Autodesk Fusion 360 part; units mm, degrees
note: some values were not read from the file. Set by a fixed rule: which sketch regions a step uses.
(part 2 of 8)
  line L93 (183.7882, -189.4826) -> (184.4852, -189.4634)
  spline S326 degree 3 poles (184.4852, -189.4634) (184.503, -190.2023) (184.6781, -192.2532) (184.527, -192.5784) knots 0 0 0 0 1 1 1 1
  spline S327 degree 3 poles (184.527, -192.5784) (183.4311, -191.7836) (182.2603, -193.7085) (183.3586, -193.8838) knots 0 0 0 0 1 1 1 1
  spline S328 degree 3 poles (183.3586, -193.8838) (183.8477, -193.9337) (184.1665, -193.9552) (184.6949, -194.0483) knots 0 0 0 0 1 1 1 1
  spline S329 degree 2 poles (184.6949, -194.0483) (184.7596, -194.5248) (184.7763, -194.8358) knots 0 0 0 1 1 1
  spline S330 degree 3 poles (184.7763, -194.8358) (183.9042, -195.3624) (183.4164, -195.9409) (183.2408, -196.7861) knots 0 0 0 0 1 1 1 1
  spline S331 degree 3 poles (183.2408, -196.7861) (183.1875, -197.6071) (183.7053, -198.7877) (184.6749, -199.0522) knots 0 0 0 0 1 1 1 1
  line L94 (184.6749, -199.0522) -> (184.423, -200.3759)
  spline S332 degree 3 poles (184.423, -200.3759) (183.7928, -200.5585) (183.5709, -200.5779) (182.9409, -200.6201) knots 0 0 0 0 1 1 1 1
  spline S333 degree 3 poles (182.9409, -200.6201) (182.6208, -200.6492) (182.7483, -200.87) (182.8157, -201.1544) knots 0 0 0 0 1 1 1 1
  spline S334 degree 3 poles (182.8157, -201.1544) (182.9162, -201.4784) (182.7891, -201.5678) (183.1468, -201.7487) knots 0 0 0 0 1 1 1 1
  spline S335 degree 3 poles (183.1468, -201.7487) (183.464, -201.8608) (183.6385, -201.9315) (183.9663, -202.1236) knots 0 0 0 0 1 1 1 1
  spline S336 degree 3 poles (183.9663, -202.1236) (183.9935, -202.4344) (183.976, -202.8518) (184.007, -203.1742) knots 0 0 0 0 1 1 1 1
  spline S337 degree 3 poles (184.007, -203.1742) (184.1755, -203.8454) (184.5886, -204.0182) (185.3208, -203.949) knots 0 0 0 0 1 1 1 1
  spline S338 degree 3 poles (185.3208, -203.949) (186.1138, -203.6409) (186.3928, -203.0862) (186.4441, -202.4283) knots 0 0 0 0 1 1 1 1
  spline S339 degree 2 poles (186.4441, -202.4283) (186.5431, -199.3372) (186.4347, -198.0017) knots 0 0 0 1 1 1
  line L95 (186.4347, -198.0017) -> (185.4047, -196.9892)
  line L96 (185.4047, -196.9892) -> (186.6001, -195.8305)
  spline S340 degree 3 poles (186.6001, -195.8305) (186.3828, -191.254) (186.2731, -187.3174) (185.6278, -182.7417) knots 0 0 0 0 1 1 1 1
  spline S341 degree 3 poles (185.6278, -182.7417) (185.4537, -182.1579) (185.066, -181.8566) (184.4242, -181.7632) knots 0 0 0 0 1 1 1 1
  spline S342 degree 3 poles (160.4078, -156.8007) (157.9023, -157.1956) (155.5538, -158.6101) (153.958, -160.6852) knots 0 0 0 0 1 1 1 1
  spline S343 degree 3 poles (153.958, -160.6852) (152.3623, -162.7604) (151.535, -165.476) (151.686, -168.1431) knots 0 0 0 0 1 1 1 1
  spline S344 degree 3 poles (151.686, -168.1431) (151.829, -170.6692) (152.8449, -173.1304) (154.5006, -174.962) knots 0 0 0 0 1 1 1 1
  spline S345 degree 3 poles (154.5006, -174.962) (156.1564, -176.7936) (158.4388, -177.9812) (160.8245, -178.2524) knots 0 0 0 0 1 1 1 1
  line L97 (160.8245, -178.2524) -> (169.7689, -178.3081)
  spline S346 degree 3 poles (169.7689, -178.3081) (173.9803, -176.478) (178.5319, -175.5232) (183.0868, -175.5142) knots 0 0 0 0 1 1 1 1
  spline S347 degree 3 poles (183.0868, -175.5142) (188.9607, -175.5026) (194.8313, -177.0765) (199.9869, -180.0452) knots 0 0 0 0 1 1 1 1
  line L98 (199.9869, -180.0452) -> (207.8706, -180.5328)
  spline S348 degree 3 poles (207.8706, -180.5328) (210.513, -180.3699) (213.0767, -179.0716) (214.8493, -176.9985) knots 0 0 0 0 1 1 1 1
  spline S349 degree 3 poles (214.8493, -176.9985) (216.622, -174.9255) (217.5826, -172.1023) (217.4642, -169.3136) knots 0 0 0 0 1 1 1 1
  spline S350 degree 3 poles (217.4642, -169.3136) (217.3685, -167.0606) (216.5801, -164.8462) (215.246, -163.0838) knots 0 0 0 0 1 1 1 1
  spline S351 degree 3 poles (215.246, -163.0838) (213.912, -161.3214) (212.0391, -160.02) (209.9773, -159.4225) knots 0 0 0 0 1 1 1 1
  line L99 (209.9773, -159.4225) -> (201.3192, -158.7839)
  spline S352 degree 3 poles (201.3192, -158.7839) (196.2891, -161.1841) (190.713, -162.2999) (185.1988, -162.0098) knots 0 0 0 0 1 1 1 1
  spline S353 degree 3 poles (185.1988, -162.0098) (179.7817, -161.7247) (174.433, -160.084) (169.716, -157.2605) knots 0 0 0 0 1 1 1 1
  line L100 (169.716, -157.2605) -> (160.4078, -156.8007)
  spline S354 degree 3 poles (158.3675, -159.7622) (158.1166, -159.7544) (157.8633, -159.8596) (157.6892, -160.0503) knots 0 0 0 0 1 1 1 1
  spline S355 degree 3 poles (157.6892, -160.0503) (157.5151, -160.241) (157.4245, -160.5147) (157.4538, -160.7776) knots 0 0 0 0 1 1 1 1
  spline S356 degree 3 poles (157.4538, -160.7776) (157.4812, -161.0245) (157.613, -161.2554) (157.804, -161.401) knots 0 0 0 0 1 1 1 1
  spline S357 degree 3 poles (157.804, -161.401) (157.9951, -161.5465) (158.2421, -161.6059) (158.475, -161.5674) knots 0 0 0 0 1 1 1 1
  spline S358 degree 3 poles (158.475, -161.5674) (158.6793, -161.5335) (158.8726, -161.4252) (159.0102, -161.2623) knots 0 0 0 0 1 1 1 1
  spline S359 degree 3 poles (159.0102, -161.2623) (159.1479, -161.0995) (159.2281, -160.8829) (159.2275, -160.6648) knots 0 0 0 0 1 1 1 1
  spline S360 degree 3 poles (159.2275, -160.6648) (159.2267, -160.429) (159.1308, -160.1961) (158.9712, -160.0309) knots 0 0 0 0 1 1 1 1
  spline S361 degree 3 poles (158.9712, -160.0309) (158.8116, -159.8658) (158.5909, -159.7694) (158.3675, -159.7622) knots 0 0 0 0 1 1 1 1
  spline S362 degree 3 poles (157.7617, -173.0749) (157.5108, -173.0671) (157.2574, -173.1722) (157.0833, -173.363) knots 0 0 0 0 1 1 1 1
  spline S363 degree 3 poles (157.0833, -173.363) (156.9092, -173.5536) (156.8187, -173.8274) (156.8479, -174.0903) knots 0 0 0 0 1 1 1 1
  spline S364 degree 3 poles (156.8479, -174.0903) (156.8753, -174.3372) (157.0071, -174.5681) (157.1982, -174.7136) knots 0 0 0 0 1 1 1 1
  spline S365 degree 3 poles (157.1982, -174.7136) (157.3893, -174.8592) (157.6363, -174.9186) (157.8692, -174.88) knots 0 0 0 0 1 1 1 1
  spline S366 degree 3 poles (157.8692, -174.88) (158.0735, -174.8462) (158.2667, -174.7378) (158.4044, -174.575) knots 0 0 0 0 1 1 1 1
  spline S367 degree 3 poles (158.4044, -174.575) (158.542, -174.4121) (158.6223, -174.1956) (158.6216, -173.9774) knots 0 0 0 0 1 1 1 1
  spline S368 degree 3 poles (158.6216, -173.9774) (158.6209, -173.7417) (158.525, -173.5087) (158.3654, -173.3436) knots 0 0 0 0 1 1 1 1
  spline S369 degree 3 poles (158.3654, -173.3436) (158.2058, -173.1785) (157.9851, -173.0821) (157.7617, -173.0749) knots 0 0 0 0 1 1 1 1
  spline S370 degree 3 poles (174.2321, -167.2173) (173.9813, -167.2095) (173.7279, -167.3147) (173.5538, -167.5054) knots 0 0 0 0 1 1 1 1
  spline S371 degree 3 poles (173.5538, -167.5054) (173.3797, -167.6961) (173.2892, -167.9698) (173.3184, -168.2327) knots 0 0 0 0 1 1 1 1
  spline S372 degree 3 poles (173.3184, -168.2327) (173.3458, -168.4796) (173.4776, -168.7105) (173.6687, -168.856) knots 0 0 0 0 1 1 1 1
  spline S373 degree 3 poles (173.6687, -168.856) (173.8597, -169.0016) (174.1068, -169.061) (174.3396, -169.0224) knots 0 0 0 0 1 1 1 1
  spline S374 degree 3 poles (174.3396, -169.0224) (174.544, -168.9886) (174.7372, -168.8802) (174.8749, -168.7174) knots 0 0 0 0 1 1 1 1
  spline S375 degree 3 poles (174.8749, -168.7174) (175.0125, -168.5546) (175.0928, -168.338) (175.0921, -168.1199) knots 0 0 0 0 1 1 1 1
  spline S376 degree 3 poles (175.0921, -168.1199) (175.0913, -167.8841) (174.9955, -167.6511) (174.8359, -167.486) knots 0 0 0 0 1 1 1 1
  spline S377 degree 3 poles (174.8359, -167.486) (174.6763, -167.3209) (174.4556, -167.2245) (174.2321, -167.2173) knots 0 0 0 0 1 1 1 1
  spline S378 degree 3 poles (194.916, -168.2945) (194.6651, -168.2867) (194.4117, -168.3919) (194.2376, -168.5826) knots 0 0 0 0 1 1 1 1
  spline S379 degree 3 poles (194.2376, -168.5826) (194.0636, -168.7733) (193.973, -169.047) (194.0022, -169.3099) knots 0 0 0 0 1 1 1 1
  spline S380 degree 3 poles (194.0022, -169.3099) (194.0297, -169.5568) (194.1615, -169.7877) (194.3525, -169.9333) knots 0 0 0 0 1 1 1 1
  spline S381 degree 3 poles (194.3525, -169.9333) (194.5436, -170.0788) (194.7906, -170.1382) (195.0235, -170.0997) knots 0 0 0 0 1 1 1 1
  spline S382 degree 3 poles (195.0235, -170.0997) (195.2278, -170.0658) (195.4211, -169.9575) (195.5587, -169.7946) knots 0 0 0 0 1 1 1 1
  spline S383 degree 3 poles (195.5587, -169.7946) (195.6964, -169.6318) (195.7766, -169.4153) (195.776, -169.1971) knots 0 0 0 0 1 1 1 1
  spline S384 degree 3 poles (195.776, -169.1971) (195.7752, -168.9613) (195.6793, -168.7284) (195.5197, -168.5632) knots 0 0 0 0 1 1 1 1
  spline S385 degree 3 poles (195.5197, -168.5632) (195.3601, -168.3981) (195.1394, -168.3017) (194.916, -168.2945) knots 0 0 0 0 1 1 1 1
  spline S386 degree 3 poles (211.3226, -162.5043) (211.0718, -162.4965) (210.8184, -162.6017) (210.6443, -162.7924) knots 0 0 0 0 1 1 1 1
  spline S387 degree 3 poles (210.6443, -162.7924) (210.4702, -162.9831) (210.3796, -163.2568) (210.4089, -163.5197) knots 0 0 0 0 1 1 1 1
  spline S388 degree 3 poles (210.4089, -163.5197) (210.4363, -163.7666) (210.5681, -163.9975) (210.7592, -164.143) knots 0 0 0 0 1 1 1 1
  spline S389 degree 3 poles (210.7592, -164.143) (210.9502, -164.2886) (211.1973, -164.348) (211.4301, -164.3094) knots 0 0 0 0 1 1 1 1
  spline S390 degree 3 poles (211.4301, -164.3094) (211.6345, -164.2756) (211.8277, -164.1672) (211.9654, -164.0044) knots 0 0 0 0 1 1 1 1
  spline S391 degree 3 poles (211.9654, -164.0044) (212.103, -163.8415) (212.1833, -163.625) (212.1826, -163.4068) knots 0 0 0 0 1 1 1 1
  spline S392 degree 3 poles (212.1826, -163.4068) (212.1818, -163.1711) (212.0859, -162.9381) (211.9264, -162.773) knots 0 0 0 0 1 1 1 1
  spline S393 degree 3 poles (211.9264, -162.773) (211.7668, -162.6079) (211.5461, -162.5115) (211.3226, -162.5043) knots 0 0 0 0 1 1 1 1
  spline S394 degree 3 poles (210.5565, -175.768) (210.3057, -175.7602) (210.0523, -175.8654) (209.8782, -176.0561) knots 0 0 0 0 1 1 1 1
  spline S395 degree 3 poles (209.8782, -176.0561) (209.7041, -176.2468) (209.6136, -176.5205) (209.6428, -176.7834) knots 0 0 0 0 1 1 1 1
  spline S396 degree 3 poles (209.6428, -176.7834) (209.6702, -177.0303) (209.802, -177.2612) (209.9931, -177.4067) knots 0 0 0 0 1 1 1 1
  spline S397 degree 3 poles (209.9931, -177.4067) (210.1842, -177.5523) (210.4312, -177.6117) (210.6641, -177.5731) knots 0 0 0 0 1 1 1 1
  spline S398 degree 3 poles (210.6641, -177.5731) (210.8684, -177.5393) (211.0616, -177.4309) (211.1993, -177.2681) knots 0 0 0 0 1 1 1 1
  spline S399 degree 3 poles (211.1993, -177.2681) (211.3369, -177.1053) (211.4172, -176.8887) (211.4165, -176.6706) knots 0 0 0 0 1 1 1 1
  spline S400 degree 3 poles (211.4165, -176.6706) (211.4158, -176.4348) (211.3199, -176.2019) (211.1603, -176.0367) knots 0 0 0 0 1 1 1 1
  spline S401 degree 3 poles (211.1603, -176.0367) (211.0007, -175.8716) (210.78, -175.7752) (210.5565, -175.768) knots 0 0 0 0 1 1 1 1
  line L101 (197.8229, -166.7115) -> (197.8229, -165.4323)
  line L102 (197.8229, -165.4323) -> (207.3988, -165.7016)
  spline S402 degree 3 poles (207.3988, -165.7016) (208.186, -165.9883) (208.8833, -166.5431) (209.3609, -167.2627) knots 0 0 0 0 1 1 1 1
  spline S403 degree 3 poles (209.3609, -167.2627) (209.8385, -167.9823) (210.094, -168.8631) (210.0801, -169.7413) knots 0 0 0 0 1 1 1 1
  spline S404 degree 3 poles (210.0801, -169.7413) (210.0678, -170.5109) (209.85, -171.2758) (209.4581, -171.9252) knots 0 0 0 0 1 1 1 1
  spline S405 degree 3 poles (209.4581, -171.9252) (209.0663, -172.5746) (208.5016, -173.1067) (207.8457, -173.4444) knots 0 0 0 0 1 1 1 1
  line L103 (207.8457, -173.4444) -> (197.7591, -173.3097)
  line L104 (197.7591, -173.3097) -> (197.6953, -171.8958)
  line L105 (197.6953, -171.8958) -> (199.3551, -171.9631)
  line L106 (199.3551, -171.9631) -> (199.3551, -166.8462)
  line L107 (199.3551, -166.8462) -> (197.8229, -166.7115)
  line L108 (171.2386, -170.5609) -> (171.2386, -171.8224)
  line L109 (171.2386, -171.8224) -> (161.9108, -171.5568)
  spline S406 degree 3 poles (161.9108, -171.5568) (161.1419, -171.2657) (160.4633, -170.7156) (159.9986, -170.007) knots 0 0 0 0 1 1 1 1
  spline S407 degree 3 poles (159.9986, -170.007) (159.5341, -169.2983) (159.2858, -168.4344) (159.299, -167.5729) knots 0 0 0 0 1 1 1 1
  spline S408 degree 3 poles (159.299, -167.5729) (159.3107, -166.8173) (159.5222, -166.0662) (159.9036, -165.4264) knots 0 0 0 0 1 1 1 1
  spline S409 degree 3 poles (159.9036, -165.4264) (160.2849, -164.7865) (160.835, -164.2598) (161.4755, -163.9211) knots 0 0 0 0 1 1 1 1
  line L110 (161.4755, -163.9211) -> (171.3008, -164.0539)
  line L111 (171.3008, -164.0539) -> (171.3629, -165.4482)
  line L112 (171.3629, -165.4482) -> (169.7461, -165.3818)
  line L113 (169.7461, -165.3818) -> (169.7461, -170.428)
  line L114 (169.7461, -170.428) -> (171.2386, -170.5609)
  spline S410 degree 3 poles (232.2847, -186.5416) (232.1541, -186.5455) (232.023, -186.5187) (231.9078, -186.4696) knots 0 0 0 0 1 1 1 1
  spline S411 degree 3 poles (231.9078, -186.4696) (231.7926, -186.4204) (231.6934, -186.3489) (231.6165, -186.2648) knots 0 0 0 0 1 1 1 1
  spline S412 degree 3 poles (231.6165, -186.2648) (231.4626, -186.0968) (231.4012, -185.883) (231.4098, -185.6754) knots 0 0 0 0 1 1 1 1
  spline S413 degree 3 poles (231.4098, -185.6754) (231.4184, -185.4716) (231.4942, -185.2655) (231.6558, -185.1073) knots 0 0 0 0 1 1 1 1
  spline S414 degree 3 poles (231.6558, -185.1073) (231.7367, -185.0281) (231.8382, -184.9619) (231.9537, -184.9177) knots 0 0 0 0 1 1 1 1
  spline S415 degree 3 poles (231.9537, -184.9177) (232.0693, -184.8734) (232.1989, -184.8517) (232.3269, -184.8586) knots 0 0 0 0 1 1 1 1
  spline S416 degree 3 poles (232.3269, -184.8586) (232.4508, -184.8655) (232.5717, -184.899) (232.6764, -184.952) knots 0 0 0 0 1 1 1 1
  spline S417 degree 3 poles (232.6764, -184.952) (232.781, -185.0051) (232.8697, -185.0773) (232.9378, -185.1598) knots 0 0 0 0 1 1 1 1
  spline S418 degree 3 poles (232.9378, -185.1598) (233.074, -185.3249) (233.1259, -185.5276) (233.1175, -185.7249) knots 0 0 0 0 1 1 1 1
  spline S419 degree 3 poles (233.1175, -185.7249) (233.1089, -185.9178) (233.0432, -186.1128) (232.8992, -186.2682) knots 0 0 0 0 1 1 1 1
  spline S420 degree 3 poles (232.8992, -186.2682) (232.8271, -186.346) (232.7362, -186.413) (232.6309, -186.4612) knots 0 0 0 0 1 1 1 1
  spline S421 degree 3 poles (232.6309, -186.4612) (232.5257, -186.5093) (232.4061, -186.5384) (232.2847, -186.5416) knots 0 0 0 0 1 1 1 1
  line L115 (227.7328, -168.9136) -> (226.8239, -182.4454)
  spline S422 degree 3 poles (226.8239, -182.4454) (226.7937, -182.7594) (226.9079, -183.0808) (227.1399, -183.3361) knots 0 0 0 0 1 1 1 1
  spline S423 degree 3 poles (227.1399, -183.3361) (227.3655, -183.5842) (227.7008, -183.7681) (228.0728, -183.8477) knots 0 0 0 0 1 1 1 1
  line L116 (228.0728, -183.8477) -> (237.3253, -184.6143)
  spline S424 degree 3 poles (237.3253, -184.6143) (237.5012, -184.6075) (237.6747, -184.5645) (237.8245, -184.4908) knots 0 0 0 0 1 1 1 1
  spline S425 degree 3 poles (237.8245, -184.4908) (237.9742, -184.4172) (238.0999, -184.3129) (238.1862, -184.1909) knots 0 0 0 0 1 1 1 1
  spline S426 degree 3 poles (238.1862, -184.1909) (238.3383, -183.9756) (238.3647, -183.7203) (238.3912, -183.4743) knots 0 0 0 0 1 1 1 1
  spline S427 degree 3 poles (238.3912, -183.4743) (238.7635, -180.0133) (239.0915, -176.5494) (239.375, -173.0831) knots 0 0 0 0 1 1 1 1
  spline S428 degree 3 poles (239.375, -173.0831) (239.7105, -168.9816) (239.9838, -164.8768) (240.1949, -160.7701) knots 0 0 0 0 1 1 1 1
  spline S429 degree 3 poles (240.1949, -160.7701) (240.2035, -160.5623) (240.1053, -160.3532) (239.9284, -160.2) knots 0 0 0 0 1 1 1 1
  spline S430 degree 3 poles (239.9284, -160.2) (239.7458, -160.0419) (239.481, -159.9457) (239.211, -159.9394) knots 0 0 0 0 1 1 1 1
  line L117 (239.211, -159.9394) -> (229.2701, -159.4834)
  spline S431 degree 3 poles (229.2701, -159.4834) (228.9483, -159.5221) (228.6532, -159.6826) (228.4912, -159.9069) knots 0 0 0 0 1 1 1 1
  spline S432 degree 3 poles (228.4912, -159.9069) (228.3918, -160.0445) (228.3416, -160.2043) (228.3477, -160.3629) knots 0 0 0 0 1 1 1 1
  line L118 (228.3477, -160.3629) -> (228.2043, -163.0747)
  line L119 (228.2043, -163.0747) -> (227.2307, -163.0869)
  spline S433 degree 3 poles (227.2307, -163.0869) (227.1358, -163.0878) (227.0401, -163.0908) (226.9473, -163.1071) knots 0 0 0 0 1 1 1 1
  spline S434 degree 3 poles (226.9473, -163.1071) (226.8545, -163.1236) (226.7652, -163.1535) (226.6875, -163.1969) knots 0 0 0 0 1 1 1 1
  spline S435 degree 3 poles (226.6875, -163.1969) (226.5164, -163.2926) (226.4068, -163.4543) (226.4006, -163.6204) knots 0 0 0 0 1 1 1 1
  line L120 (226.4006, -163.6204) -> (226.0521, -168.1971)
  spline S436 degree 3 poles (226.0521, -168.1971) (226.0834, -168.3183) (226.1507, -168.4335) (226.247, -168.5308) knots 0 0 0 0 1 1 1 1
  spline S437 degree 3 poles (226.247, -168.5308) (226.3376, -168.6226) (226.454, -168.6982) (226.5851, -168.7508) knots 0 0 0 0 1 1 1 1
  line L121 (226.5851, -168.7508) -> (227.7328, -168.9136)
  spline S438 degree 3 poles (224.9792, -160.4081) (224.3309, -164.8353) (223.9577, -169.288) (223.8616, -173.7444) knots 0 0 0 0 1 1 1 1
  spline S439 degree 3 poles (223.8616, -173.7444) (223.7656, -178.1893) (223.8819, -182.6352) (223.9034, -187.0807) knots 0 0 0 0 1 1 1 1
  line L122 (223.9034, -187.0807) -> (224.0451, -216.3332)
  spline S440 degree 3 poles (224.0451, -216.3332) (224.0959, -216.2302) (224.1963, -216.1434) (224.3211, -216.0945) knots 0 0 0 0 1 1 1 1
  spline S441 degree 3 poles (224.3211, -216.0945) (224.4458, -216.0455) (224.5937, -216.0351) (224.7274, -216.0658) knots 0 0 0 0 1 1 1 1
  spline S442 degree 3 poles (224.7274, -216.0658) (224.8788, -216.1005) (225.0075, -216.1858) (225.0933, -216.2909) knots 0 0 0 0 1 1 1 1
  spline S443 degree 3 poles (225.0933, -216.2909) (225.1791, -216.396) (225.2241, -216.5197) (225.2408, -216.6442) knots 0 0 0 0 1 1 1 1
  spline S444 degree 3 poles (225.2408, -216.6442) (225.2743, -216.8932) (225.199, -217.1423) (225.1693, -217.3916) knots 0 0 0 0 1 1 1 1
  spline S445 degree 3 poles (225.1693, -217.3916) (225.0952, -218.013) (225.3157, -218.6538) (225.7774, -219.1588) knots 0 0 0 0 1 1 1 1
  spline S446 degree 3 poles (225.7774, -219.1588) (225.815, -218.9656) (225.981, -218.7912) (226.2048, -218.71) knots 0 0 0 0 1 1 1 1
  spline S447 degree 3 poles (226.2048, -218.71) (226.4285, -218.6288) (226.7031, -218.6432) (226.9115, -218.7472) knots 0 0 0 0 1 1 1 1
  spline S448 degree 3 poles (226.9115, -218.7472) (227.0213, -218.8019) (227.1119, -218.8791) (227.1826, -218.9655) knots 0 0 0 0 1 1 1 1
  spline S449 degree 3 poles (227.1826, -218.9655) (227.2533, -219.0519) (227.3047, -219.1476) (227.3452, -219.2455) knots 0 0 0 0 1 1 1 1
  spline S450 degree 3 poles (227.3452, -219.2455) (227.4261, -219.4413) (227.4646, -219.6471) (227.5475, -219.8424) knots 0 0 0 0 1 1 1 1
  spline S451 degree 3 poles (227.5475, -219.8424) (227.7556, -220.3325) (228.256, -220.7385) (228.8682, -220.9141) knots 0 0 0 0 1 1 1 1
  spline S452 degree 3 poles (228.8682, -220.9141) (228.7957, -220.6987) (228.8134, -220.4647) (228.9179, -220.2577) knots 0 0 0 0 1 1 1 1
  spline S453 degree 3 poles (228.9179, -220.2577) (229.0225, -220.0507) (229.2131, -219.8719) (229.4528, -219.756) knots 0 0 0 0 1 1 1 1
  spline S454 degree 3 poles (229.4528, -219.756) (229.7406, -219.6168) (230.1051, -219.5715) (230.4233, -219.6593) knots 0 0 0 0 1 1 1 1
  spline S455 degree 3 poles (230.4233, -219.6593) (230.6504, -219.722) (230.8475, -219.8507) (230.9689, -220.0156) knots 0 0 0 0 1 1 1 1
  spline S456 degree 3 poles (230.9689, -220.0156) (231.0903, -220.1804) (231.135, -220.38) (231.0926, -220.568) knots 0 0 0 0 1 1 1 1
  spline S457 degree 3 poles (231.0926, -220.568) (231.4741, -220.5281) (231.8292, -220.3496) (232.038, -220.0927) knots 0 0 0 0 1 1 1 1
  spline S458 degree 3 poles (232.038, -220.0927) (232.2522, -219.8293) (232.3081, -219.5075) (232.4059, -219.2037) knots 0 0 0 0 1 1 1 1
  spline S459 degree 3 poles (232.4059, -219.2037) (232.4547, -219.0518) (232.5158, -218.9011) (232.6125, -218.7644) knots 0 0 0 0 1 1 1 1
  spline S460 degree 3 poles (232.6125, -218.7644) (232.7092, -218.6277) (232.8438, -218.5051) (233.0157, -218.428) knots 0 0 0 0 1 1 1 1
  spline S461 degree 3 poles (233.0157, -218.428) (233.2451, -218.325) (233.5351, -218.312) (233.7777, -218.3938) knots 0 0 0 0 1 1 1 1
  spline S462 degree 3 poles (233.7777, -218.3938) (234.0202, -218.4756) (234.2099, -218.6505) (234.276, -218.8532) knots 0 0 0 0 1 1 1 1
  spline S463 degree 3 poles (234.276, -218.8532) (234.4984, -218.5712) (234.5834, -218.2226) (234.5096, -217.895) knots 0 0 0 0 1 1 1 1
  spline S464 degree 3 poles (234.5096, -217.895) (234.4459, -217.6125) (234.272, -217.3547) (234.1237, -217.093) knots 0 0 0 0 1 1 1 1
  spline S465 degree 3 poles (234.1237, -217.093) (233.9753, -216.8312) (233.8485, -216.5484) (233.8884, -216.263) knots 0 0 0 0 1 1 1 1
  spline S466 degree 3 poles (233.8884, -216.263) (233.9241, -216.0072) (234.0999, -215.7657) (234.3612, -215.6135) knots 0 0 0 0 1 1 1 1
  spline S467 degree 3 poles (234.3612, -215.6135) (234.6226, -215.4614) (234.9654, -215.401) (235.2831, -215.451) knots 0 0 0 0 1 1 1 1
  spline S468 degree 3 poles (235.2831, -215.451) (235.3402, -215.1074) (235.1906, -214.7457) (234.888, -214.496) knots 0 0 0 0 1 1 1 1
  spline S469 degree 3 poles (234.888, -214.496) (234.7354, -214.3702) (234.5495, -214.2736) (234.3674, -214.1756) knots 0 0 0 0 1 1 1 1
  spline S470 degree 3 poles (234.3674, -214.1756) (234.1853, -214.0776) (234.0031, -213.9754) (233.8619, -213.8414) knots 0 0 0 0 1 1 1 1
  spline S471 degree 3 poles (233.8619, -213.8414) (233.7252, -213.7114) (233.6308, -213.5535) (233.5906, -213.3872) knots 0 0 0 0 1 1 1 1
  spline S472 degree 3 poles (233.5906, -213.3872) (233.5503, -213.2208) (233.5643, -213.0464) (233.6307, -212.8854) knots 0 0 0 0 1 1 1 1
  spline S473 degree 3 poles (233.6307, -212.8854) (233.6971, -212.7244) (233.8159, -212.5773) (233.9723, -212.4622) knots 0 0 0 0 1 1 1 1
  spline S474 degree 3 poles (233.9723, -212.4622) (234.1287, -212.347) (234.3224, -212.2642) (234.5294, -212.2238) knots 0 0 0 0 1 1 1 1
  spline S475 degree 3 poles (234.5294, -212.2238) (234.4537, -212.0526) (234.3633, -211.8854) (234.259, -211.7239) knots 0 0 0 0 1 1 1 1
  spline S476 degree 3 poles (234.259, -211.7239) (233.6061, -210.7129) (232.4306, -209.9506) (231.8561, -208.91) knots 0 0 0 0 1 1 1 1
  spline S477 degree 3 poles (231.8561, -208.91) (231.3602, -208.0116) (231.3617, -206.9812) (231.6087, -206.02) knots 0 0 0 0 1 1 1 1
  spline S478 degree 3 poles (231.6087, -206.02) (231.8556, -205.0587) (232.3335, -204.1467) (232.7708, -203.2292) knots 0 0 0 0 1 1 1 1
  spline S479 degree 3 poles (232.7708, -203.2292) (233.5372, -201.6216) (234.1852, -199.9804) (234.8773, -198.3516) knots 0 0 0 0 1 1 1 1
  spline S480 degree 3 poles (234.8773, -198.3516) (236.5894, -194.3226) (238.5767, -190.3562) (239.8247, -186.221) knots 0 0 0 0 1 1 1 1
  spline S481 degree 3 poles (239.8247, -186.221) (240.7522, -183.1475) (241.2637, -180.0038) (241.6284, -176.8565) knots 0 0 0 0 1 1 1 1
  spline S482 degree 3 poles (241.6284, -176.8565) (242.2674, -171.3418) (242.46, -165.7944) (242.2047, -160.2601) knots 0 0 0 0 1 1 1 1
  spline S483 degree 3 poles (242.2047, -160.2601) (241.9853, -158.8939) (241.2361, -157.5845) (240.0848, -156.555) knots 0 0 0 0 1 1 1 1
  spline S484 degree 3 poles (240.0848, -156.555) (238.9335, -155.5256) (237.385, -154.7805) (235.7034, -154.4469) knots 0 0 0 0 1 1 1 1
  spline S485 degree 3 poles (235.7034, -154.4469) (233.3054, -153.9711) (230.6576, -154.3602) (228.6323, -155.4859) knots 0 0 0 0 1 1 1 1
  spline S486 degree 3 poles (228.6323, -155.4859) (226.607, -156.6116) (225.239, -158.4547) (224.9792, -160.4081) knots 0 0 0 0 1 1 1 1
  spline S487 degree 3 poles (229.6681, -216.0195) (229.5156, -216.0234) (229.3626, -215.991) (229.2301, -215.9308) knots 0 0 0 0 1 1 1 1
  spline S488 degree 3 poles (229.2301, -215.9308) (229.0976, -215.8707) (228.9853, -215.7838) (228.9, -215.6833) knots 0 0 0 0 1 1 1 1
  spline S489 degree 3 poles (228.9, -215.6833) (228.7293, -215.4821) (228.6691, -215.2317) (228.6794, -214.9893) knots 0 0 0 0 1 1 1 1
  spline S490 degree 3 poles (228.6794, -214.9893) (228.6892, -214.7522) (228.7668, -214.5112) (228.9465, -214.3218) knots 0 0 0 0 1 1 1 1
  spline S491 degree 3 poles (228.9465, -214.3218) (229.0363, -214.2271) (229.151, -214.1466) (229.2836, -214.0922) knots 0 0 0 0 1 1 1 1
  spline S492 degree 3 poles (229.2836, -214.0922) (229.4162, -214.0378) (229.5669, -214.01) (229.7158, -214.0178) knots 0 0 0 0 1 1 1 1
  spline S493 degree 3 poles (229.7158, -214.0178) (229.8608, -214.0256) (230.0019, -214.0667) (230.1224, -214.1313) knots 0 0 0 0 1 1 1 1
  spline S494 degree 3 poles (230.1224, -214.1313) (230.2429, -214.1958) (230.343, -214.2832) (230.4184, -214.3819) knots 0 0 0 0 1 1 1 1
  spline S495 degree 3 poles (230.4184, -214.3819) (230.5692, -214.5794) (230.6192, -214.8173) (230.6092, -215.0481) knots 0 0 0 0 1 1 1 1
  spline S496 degree 3 poles (230.6092, -215.0481) (230.5994, -215.2731) (230.5327, -215.5016) (230.3729, -215.6875) knots 0 0 0 0 1 1 1 1
  spline S497 degree 3 poles (230.3729, -215.6875) (230.293, -215.7804) (230.1903, -215.8617) (230.0696, -215.9205) knots 0 0 0 0 1 1 1 1
  spline S498 degree 3 poles (230.0696, -215.9205) (229.9488, -215.9794) (229.8097, -216.0154) (229.6681, -216.0195) knots 0 0 0 0 1 1 1 1
  spline S499 degree 3 poles (234.7196, -158.8094) (234.5889, -158.8133) (234.4578, -158.7865) (234.3427, -158.7374) knots 0 0 0 0 1 1 1 1
  spline S500 degree 3 poles (234.3427, -158.7374) (234.2274, -158.6882) (234.1283, -158.6166) (234.0513, -158.5326) knots 0 0 0 0 1 1 1 1
  spline S501 degree 3 poles (234.0513, -158.5326) (233.8975, -158.3646) (233.8361, -158.1508) (233.8447, -157.9431) knots 0 0 0 0 1 1 1 1
  spline S502 degree 3 poles (233.8447, -157.9431) (233.8532, -157.7394) (233.9291, -157.5333) (234.0907, -157.3751) knots 0 0 0 0 1 1 1 1
  spline S503 degree 3 poles (234.0907, -157.3751) (234.1716, -157.2959) (234.273, -157.2297) (234.3886, -157.1855) knots 0 0 0 0 1 1 1 1
  spline S504 degree 3 poles (234.3886, -157.1855) (234.5042, -157.1412) (234.6338, -157.1195) (234.7617, -157.1264) knots 0 0 0 0 1 1 1 1
  spline S505 degree 3 poles (234.7617, -157.1264) (234.8857, -157.1332) (235.0065, -157.1668) (235.1112, -157.2198) knots 0 0 0 0 1 1 1 1
  spline S506 degree 3 poles (235.1112, -157.2198) (235.2159, -157.2728) (235.3046, -157.3451) (235.3727, -157.4276) knots 0 0 0 0 1 1 1 1
  spline S507 degree 3 poles (235.3727, -157.4276) (235.5089, -157.5927) (235.5608, -157.7954) (235.5524, -157.9927) knots 0 0 0 0 1 1 1 1
  spline S508 degree 3 poles (235.5524, -157.9927) (235.5438, -158.1856) (235.4781, -158.3806) (235.334, -158.536) knots 0 0 0 0 1 1 1 1
  spline S509 degree 3 poles (235.334, -158.536) (235.262, -158.6137) (235.1711, -158.6808) (235.0658, -158.7289) knots 0 0 0 0 1 1 1 1
  spline S510 degree 3 poles (235.0658, -158.7289) (234.9605, -158.7771) (234.841, -158.8062) (234.7196, -158.8094) knots 0 0 0 0 1 1 1 1
  spline S511 degree 3 poles (227.6647, -200.8911) (227.6822, -201.053) (227.7758, -201.2092) (227.9231, -201.3219) knots 0 0 0 0 1 1 1 1
  spline S512 degree 3 poles (227.9231, -201.3219) (228.0705, -201.4346) (228.2704, -201.503) (228.4747, -201.5106) knots 0 0 0 0 1 1 1 1
  spline S513 degree 3 poles (228.4747, -201.5106) (228.6537, -201.5174) (228.8349, -201.4777) (228.9845, -201.3993) knots 0 0 0 0 1 1 1 1
  spline S514 degree 3 poles (228.9845, -201.3993) (229.134, -201.3209) (229.2511, -201.204) (229.3138, -201.0706) knots 0 0 0 0 1 1 1 1
  line L123 (229.3138, -201.0706) -> (234.7342, -188.9506)
  spline S515 degree 3 poles (234.7342, -188.9506) (234.7721, -188.7798) (234.733, -188.5987) (234.6256, -188.4476) knots 0 0 0 0 1 1 1 1
  spline S516 degree 3 poles (234.6256, -188.4476) (234.5132, -188.2896) (234.3268, -188.1657) (234.1111, -188.1059) knots 0 0 0 0 1 1 1 1
  line L124 (234.1111, -188.1059) -> (228.6359, -187.6731)
  spline S517 degree 3 poles (228.6359, -187.6731) (228.4463, -187.6809) (228.2597, -187.7295) (228.1012, -187.8125) knots 0 0 0 0 1 1 1 1
  spline S518 degree 3 poles (228.1012, -187.8125) (227.8372, -187.9506) (227.6573, -188.1858) (227.6245, -188.4356) knots 0 0 0 0 1 1 1 1
  line L125 (227.6245, -188.4356) -> (227.6647, -200.8911)
  spline S519 degree 2 poles (42.3005, -37.3478) (44.6824, -37.1986) (46.1609, -37.3764) knots 0 0 0 1 1 1
  spline S520 degree 3 poles (46.1609, -37.3764) (46.1486, -38.9828) (46.0222, -41.0715) (46.5588, -41.5968) knots 0 0 0 0 1 1 1 1
  spline S521 degree 3 poles (46.5588, -41.5968) (47.2982, -42.5297) (49.4757, -43.7621) (51.7758, -43.6087) knots 0 0 0 0 1 1 1 1
  spline S522 degree 3 poles (51.7758, -43.6087) (54.1849, -43.4481) (55.5485, -41.4539) (56.4135, -39.8373) knots 0 0 0 0 1 1 1 1
  spline S523 degree 3 poles (56.4135, -39.8373) (56.9883, -38.763) (57.0364, -37.2644) (56.5452, -36.3376) knots 0 0 0 0 1 1 1 1
  spline S524 degree 3 poles (56.5452, -36.3376) (55.3223, -34.0302) (51.1006, -30.6279) (49.2623, -30.5851) knots 0 0 0 0 1 1 1 1
  spline S525 degree 3 poles (49.2623, -30.5851) (48.1099, -30.5565) (47.0647, -32.7511) (46.6652, -32.6733) knots 0 0 0 0 1 1 1 1
  spline S526 degree 3 poles (46.6652, -32.6733) (46.1984, -32.5825) (45.8739, -32.2086) (45.6209, -31.8842) knots 0 0 0 0 1 1 1 1
  spline S527 degree 3 poles (45.6209, -31.8842) (45.3133, -31.4897) (47.8314, -29.4071) (47.9152, -28.7752) knots 0 0 0 0 1 1 1 1
  spline S528 degree 3 poles (47.9152, -28.7752) (47.9918, -28.1978) (47.8113, -27.8216) (47.6419, -27.6768) knots 0 0 0 0 1 1 1 1
  spline S529 degree 3 poles (47.6419, -27.6768) (47.3081, -27.3915) (46.6155, -27.1308) (46.2177, -27.1892) knots 0 0 0 0 1 1 1 1
  spline S530 degree 3 poles (46.2177, -27.1892) (46.097, -27.2055) (45.9615, -27.278) (45.9305, -27.3722) knots 0 0 0 0 1 1 1 1
  spline S531 degree 2 poles (45.9305, -27.3722) (45.8704, -27.5548) (45.8649, -28.602) knots 0 0 0 1 1 1
  line L126 (45.8649, -28.602) -> (42.3388, -28.6884)
  spline S532 degree 2 poles (42.3388, -28.6884) (42.268, -27.792) (42.111, -27.3097) knots 0 0 0 1 1 1
  spline S533 degree 3 poles (42.111, -27.3097) (42.0729, -27.1923) (41.9082, -27.1002) (41.758, -27.0774) knots 0 0 0 0 1 1 1 1
  spline S534 degree 3 poles (41.758, -27.0774) (41.5245, -27.0407) (40.8133, -27.2978) (40.5519, -27.5954) knots 0 0 0 0 1 1 1 1
  spline S535 degree 3 poles (40.5519, -27.5954) (40.3041, -27.8775) (40.3431, -28.2758) (40.3669, -28.6165) knots 0 0 0 0 1 1 1 1
  spline S536 degree 3 poles (40.3669, -28.6165) (40.4121, -29.2648) (43.1815, -31.484) (42.9298, -31.8281) knots 0 0 0 0 1 1 1 1
  spline S537 degree 2 poles (42.9298, -31.8281) (42.6653, -32.1896) (41.8415, -32.7378) knots 0 0 0 1 1 1
  spline S538 degree 2 poles (41.8415, -32.7378) (40.3774, -30.4901) (39.2201, -30.5172) knots 0 0 0 1 1 1
  spline S539 degree 3 poles (39.2201, -30.5172) (38.2626, -30.5416) (33.464, -34.0591) (32.5579, -35.7105) knots 0 0 0 0 1 1 1 1
  spline S540 degree 3 poles (32.5579, -35.7105) (31.3288, -37.9506) (32.5601, -39.9388) (33.1023, -40.7563) knots 0 0 0 0 1 1 1 1
  spline S541 degree 3 poles (33.1023, -40.7563) (33.3794, -41.1741) (35.2288, -43.5448) (37.8476, -43.5502) knots 0 0 0 0 1 1 1 1
  spline S542 degree 3 poles (37.8476, -43.5502) (40.1414, -43.2845) (41.4973, -42.2844) (42.1259, -41.8129) knots 0 0 0 0 1 1 1 1
  spline S543 degree 3 poles (42.1259, -41.8129) (42.7128, -41.3728) (42.3083, -39.3859) (42.3004, -37.3474) knots 0 0 0 0 1 1 1 1
  line L127 (42.3004, -37.3474) -> (42.3005, -37.3478)
  spline S544 degree 3 poles (38.3941, -32.5465) (38.1404, -32.5434) (37.8541, -32.7718) (37.8558, -32.9725) knots 0 0 0 0 1 1 1 1
  spline S545 degree 3 poles (37.8558, -32.9725) (37.8575, -33.1719) (38.1452, -33.3912) (38.3969, -33.3892) knots 0 0 0 0 1 1 1 1
  spline S546 degree 3 poles (38.3969, -33.3892) (38.6397, -33.3873) (38.9061, -33.1712) (38.909, -32.9789) knots 0 0 0 0 1 1 1 1
  spline S547 degree 3 poles (38.909, -32.9789) (38.9119, -32.7809) (38.6444, -32.5494) (38.3941, -32.5465) knots 0 0 0 0 1 1 1 1
  spline S548 degree 3 poles (40.6279, -34.9239) (40.3742, -34.9208) (40.0879, -35.1492) (40.0896, -35.3499) knots 0 0 0 0 1 1 1 1
  spline S549 degree 3 poles (40.0896, -35.3499) (40.0913, -35.5493) (40.379, -35.7686) (40.6307, -35.7666) knots 0 0 0 0 1 1 1 1
  spline S550 degree 3 poles (40.6307, -35.7666) (40.8735, -35.7647) (41.1399, -35.5486) (41.1428, -35.3563) knots 0 0 0 0 1 1 1 1
  spline S551 degree 3 poles (41.1428, -35.3563) (41.1457, -35.1583) (40.8782, -34.9268) (40.6279, -34.9239) knots 0 0 0 0 1 1 1 1
  spline S552 degree 3 poles (38.3124, -34.8806) (38.0587, -34.8775) (37.7724, -35.106) (37.7741, -35.3067) knots 0 0 0 0 1 1 1 1
  spline S553 degree 3 poles (37.7741, -35.3067) (37.7758, -35.506) (38.0635, -35.7254) (38.3152, -35.7234) knots 0 0 0 0 1 1 1 1
  spline S554 degree 3 poles (38.3152, -35.7234) (38.558, -35.7215) (38.8244, -35.5054) (38.8273, -35.3131) knots 0 0 0 0 1 1 1 1
  spline S555 degree 3 poles (38.8273, -35.3131) (38.8302, -35.115) (38.5627, -34.8836) (38.3124, -34.8806) knots 0 0 0 0 1 1 1 1
  spline S556 degree 3 poles (35.8335, -34.6429) (35.5797, -34.6398) (35.2934, -34.8683) (35.2951, -35.069) knots 0 0 0 0 1 1 1 1
  spline S557 degree 3 poles (35.2951, -35.069) (35.2968, -35.2683) (35.5845, -35.4877) (35.8362, -35.4857) knots 0 0 0 0 1 1 1 1
  spline S558 degree 3 poles (35.8362, -35.4857) (36.079, -35.4838) (36.3454, -35.2677) (36.3483, -35.0754) knots 0 0 0 0 1 1 1 1
  spline S559 degree 3 poles (36.3483, -35.0754) (36.3512, -34.8773) (36.0837, -34.6459) (35.8335, -34.6429) knots 0 0 0 0 1 1 1 1
  spline S560 degree 3 poles (36.2966, -37.6687) (36.0428, -37.6657) (35.7565, -37.8941) (35.7582, -38.0948) knots 0 0 0 0 1 1 1 1
  spline S561 degree 3 poles (35.7582, -38.0948) (35.7599, -38.2942) (36.0476, -38.5135) (36.2993, -38.5115) knots 0 0 0 0 1 1 1 1
  spline S562 degree 3 poles (36.2993, -38.5115) (36.5421, -38.5097) (36.8085, -38.2935) (36.8114, -38.1013) knots 0 0 0 0 1 1 1 1
  spline S563 degree 3 poles (36.8114, -38.1013) (36.8143, -37.9032) (36.5468, -37.6717) (36.2966, -37.6687) knots 0 0 0 0 1 1 1 1
  spline S564 degree 3 poles (38.5848, -37.7119) (38.3311, -37.7088) (38.0448, -37.9373) (38.0465, -38.138) knots 0 0 0 0 1 1 1 1
  spline S565 degree 3 poles (38.0465, -38.138) (38.0482, -38.3373) (38.3359, -38.5567) (38.5876, -38.5547) knots 0 0 0 0 1 1 1 1
  spline S566 degree 3 poles (38.5876, -38.5547) (38.8304, -38.5528) (39.0968, -38.3367) (39.0997, -38.1444) knots 0 0 0 0 1 1 1 1
  spline S567 degree 3 poles (39.0997, -38.1444) (39.1026, -37.9463) (38.8351, -37.7148) (38.5848, -37.7119) knots 0 0 0 0 1 1 1 1
  spline S568 degree 3 poles (41.0093, -37.5174) (40.7556, -37.5143) (40.4693, -37.7428) (40.471, -37.9435) knots 0 0 0 0 1 1 1 1
  spline S569 degree 3 poles (40.471, -37.9435) (40.4727, -38.1429) (40.7604, -38.3622) (41.0121, -38.3602) knots 0 0 0 0 1 1 1 1
  spline S570 degree 3 poles (41.0121, -38.3602) (41.2549, -38.3583) (41.5213, -38.1422) (41.5242, -37.9499) knots 0 0 0 0 1 1 1 1
  spline S571 degree 3 poles (41.5242, -37.9499) (41.5271, -37.7519) (41.2596, -37.5204) (41.0093, -37.5174) knots 0 0 0 0 1 1 1 1
  spline S572 degree 3 poles (34.0355, -37.2148) (33.7817, -37.2117) (33.4954, -37.4401) (33.4972, -37.6409) knots 0 0 0 0 1 1 1 1
  spline S573 degree 3 poles (33.4972, -37.6409) (33.4989, -37.8402) (33.7866, -38.0596) (34.0382, -38.0576) knots 0 0 0 0 1 1 1 1
  spline S574 degree 3 poles (34.0382, -38.0576) (34.2811, -38.0557) (34.5475, -37.8395) (34.5504, -37.6473) knots 0 0 0 0 1 1 1 1
  spline S575 degree 3 poles (34.5504, -37.6473) (34.5532, -37.4492) (34.2857, -37.2177) (34.0355, -37.2148) knots 0 0 0 0 1 1 1 1
  spline S576 degree 3 poles (35.8062, -40.3703) (35.5524, -40.3673) (35.2661, -40.5957) (35.2679, -40.7964) knots 0 0 0 0 1 1 1 1
  spline S577 degree 3 poles (35.2679, -40.7964) (35.2696, -40.9957) (35.5573, -41.2151) (35.8089, -41.2131) knots 0 0 0 0 1 1 1 1
  spline S578 degree 3 poles (35.8089, -41.2131) (36.0518, -41.2112) (36.3182, -40.9951) (36.321, -40.8028) knots 0 0 0 0 1 1 1 1
  spline S579 degree 3 poles (36.321, -40.8028) (36.3239, -40.6047) (36.0564, -40.3732) (35.8062, -40.3703) knots 0 0 0 0 1 1 1 1
  spline S580 degree 3 poles (37.931, -40.3487) (37.6773, -40.3456) (37.391, -40.5741) (37.3927, -40.7748) knots 0 0 0 0 1 1 1 1
  spline S581 degree 3 poles (37.3927, -40.7748) (37.3944, -40.9742) (37.6821, -41.1935) (37.9338, -41.1915) knots 0 0 0 0 1 1 1 1
  spline S582 degree 3 poles (37.9338, -41.1915) (38.1766, -41.1896) (38.443, -40.9735) (38.4459, -40.7812) knots 0 0 0 0 1 1 1 1
  spline S583 degree 3 poles (38.4459, -40.7812) (38.4488, -40.5831) (38.1813, -40.3517) (37.931, -40.3487) knots 0 0 0 0 1 1 1 1
  spline S584 degree 3 poles (40.3555, -39.9597) (40.1018, -39.9566) (39.8155, -40.185) (39.8172, -40.3857) knots 0 0 0 0 1 1 1 1
  spline S585 degree 3 poles (39.8172, -40.3857) (39.8189, -40.5851) (40.1066, -40.8044) (40.3583, -40.8024) knots 0 0 0 0 1 1 1 1
  spline S586 degree 3 poles (40.3583, -40.8024) (40.6011, -40.8005) (40.8675, -40.5844) (40.8704, -40.3921) knots 0 0 0 0 1 1 1 1
  spline S587 degree 3 poles (40.8704, -40.3921) (40.8733, -40.1941) (40.6058, -39.9626) (40.3555, -39.9597) knots 0 0 0 0 1 1 1 1
  spline S588 degree 3 poles (49.8356, -32.568) (49.5818, -32.565) (49.2955, -32.7934) (49.2973, -32.9942) knots 0 0 0 0 1 1 1 1
  spline S589 degree 3 poles (49.2973, -32.9942) (49.2989, -33.1935) (49.5867, -33.4129) (49.8383, -33.4109) knots 0 0 0 0 1 1 1 1
  spline S590 degree 3 poles (49.8383, -33.4109) (50.0812, -33.4089) (50.3475, -33.1928) (50.3504, -33.0006) knots 0 0 0 0 1 1 1 1
  spline S591 degree 3 poles (50.3504, -33.0006) (50.3533, -32.8025) (50.0858, -32.571) (49.8356, -32.568) knots 0 0 0 0 1 1 1 1
  spline S592 degree 3 poles (47.4928, -34.859) (47.239, -34.8559) (46.9527, -35.0844) (46.9545, -35.2851) knots 0 0 0 0 1 1 1 1
  spline S593 degree 3 poles (46.9545, -35.2851) (46.9562, -35.4844) (47.2439, -35.7038) (47.4955, -35.7018) knots 0 0 0 0 1 1 1 1
  spline S594 degree 3 poles (47.4955, -35.7018) (47.7384, -35.6998) (48.0048, -35.4837) (48.0076, -35.2915) knots 0 0 0 0 1 1 1 1
  spline S595 degree 3 poles (48.0076, -35.2915) (48.0106, -35.0934) (47.743, -34.8619) (47.4928, -34.859) knots 0 0 0 0 1 1 1 1
  spline S596 degree 3 poles (49.9173, -34.8806) (49.6635, -34.8775) (49.3772, -35.106) (49.379, -35.3067) knots 0 0 0 0 1 1 1 1
  spline S597 degree 3 poles (49.379, -35.3067) (49.3806, -35.506) (49.6684, -35.7254) (49.92, -35.7234) knots 0 0 0 0 1 1 1 1
  spline S598 degree 3 poles (49.92, -35.7234) (50.1629, -35.7215) (50.4292, -35.5054) (50.4321, -35.3131) knots 0 0 0 0 1 1 1 1
  spline S599 degree 3 poles (50.4321, -35.3131) (50.435, -35.115) (50.1675, -34.8836) (49.9173, -34.8806) knots 0 0 0 0 1 1 1 1
  spline S600 degree 3 poles (52.0421, -34.6861) (51.7884, -34.683) (51.5021, -34.9115) (51.5038, -35.1122) knots 0 0 0 0 1 1 1 1
  spline S601 degree 3 poles (51.5038, -35.1122) (51.5055, -35.3115) (51.7932, -35.5309) (52.0448, -35.5289) knots 0 0 0 0 1 1 1 1
  spline S602 degree 3 poles (52.0448, -35.5289) (52.2877, -35.5269) (52.5541, -35.3108) (52.557, -35.1186) knots 0 0 0 0 1 1 1 1
  spline S603 degree 3 poles (52.557, -35.1186) (52.5598, -34.9205) (52.2924, -34.689) (52.0421, -34.6861) knots 0 0 0 0 1 1 1 1
  spline S604 degree 3 poles (47.3021, -37.4742) (47.0483, -37.4711) (46.762, -37.6995) (46.7638, -37.9002) knots 0 0 0 0 1 1 1 1
  spline S605 degree 3 poles (46.7638, -37.9002) (46.7655, -38.0996) (47.0532, -38.3189) (47.3048, -38.3169) knots 0 0 0 0 1 1 1 1
  spline S606 degree 3 poles (47.3048, -38.3169) (47.5477, -38.315) (47.8141, -38.0989) (47.817, -37.9067) knots 0 0 0 0 1 1 1 1
  spline S607 degree 3 poles (47.817, -37.9067) (47.8198, -37.7086) (47.5523, -37.4771) (47.3021, -37.4742) knots 0 0 0 0 1 1 1 1
  spline S608 degree 3 poles (47.8742, -39.7868) (47.6204, -39.7837) (47.3341, -40.0121) (47.3358, -40.2128) knots 0 0 0 0 1 1 1 1
  spline S609 degree 3 poles (47.3358, -40.2128) (47.3375, -40.4122) (47.6253, -40.6315) (47.8769, -40.6295) knots 0 0 0 0 1 1 1 1
  spline S610 degree 3 poles (47.8769, -40.6295) (48.1197, -40.6276) (48.3861, -40.4115) (48.389, -40.2193) knots 0 0 0 0 1 1 1 1
  spline S611 degree 3 poles (48.389, -40.2193) (48.3919, -40.0212) (48.1244, -39.7897) (47.8742, -39.7868) knots 0 0 0 0 1 1 1 1
  spline S612 degree 3 poles (49.7266, -37.6903) (49.4729, -37.6872) (49.1865, -37.9157) (49.1883, -38.1164) knots 0 0 0 0 1 1 1 1
  spline S613 degree 3 poles (49.1883, -38.1164) (49.19, -38.3158) (49.4777, -38.5351) (49.7293, -38.5331) knots 0 0 0 0 1 1 1 1
  spline S614 degree 3 poles (49.7293, -38.5331) (49.9722, -38.5312) (50.2386, -38.3151) (50.2415, -38.1228) knots 0 0 0 0 1 1 1 1
  spline S615 degree 3 poles (50.2415, -38.1228) (50.2443, -37.9247) (49.9768, -37.6933) (49.7266, -37.6903) knots 0 0 0 0 1 1 1 1
  spline S616 degree 3 poles (49.7266, -37.6903) (49.4729, -37.6872) (49.1865, -37.9157) (49.1883, -38.1164) knots 0 0 0 0 1 1 1 1
  spline S617 degree 3 poles (49.1883, -38.1164) (49.19, -38.3158) (49.4777, -38.5351) (49.7293, -38.5331) knots 0 0 0 0 1 1 1 1
  spline S618 degree 3 poles (49.7293, -38.5331) (49.9722, -38.5312) (50.2386, -38.3151) (50.2415, -38.1228) knots 0 0 0 0 1 1 1 1
  spline S619 degree 3 poles (50.2415, -38.1228) (50.2443, -37.9247) (49.9768, -37.6933) (49.7266, -37.6903) knots 0 0 0 0 1 1 1 1
  spline S620 degree 3 poles (50.0535, -40.4783) (49.7997, -40.4753) (49.5134, -40.7037) (49.5152, -40.9045) knots 0 0 0 0 1 1 1 1
  spline S621 degree 3 poles (49.5152, -40.9045) (49.5169, -41.1038) (49.8046, -41.3232) (50.0562, -41.3212) knots 0 0 0 0 1 1 1 1
  spline S622 degree 3 poles (50.0562, -41.3212) (50.2991, -41.3193) (50.5655, -41.1031) (50.5684, -40.9109) knots 0 0 0 0 1 1 1 1
  spline S623 degree 3 poles (50.5684, -40.9109) (50.5713, -40.7128) (50.3037, -40.4813) (50.0535, -40.4783) knots 0 0 0 0 1 1 1 1
  spline S624 degree 3 poles (52.587, -40.4568) (52.3332, -40.4537) (52.0469, -40.6822) (52.0486, -40.8829) knots 0 0 0 0 1 1 1 1
  spline S625 degree 3 poles (52.0486, -40.8829) (52.0503, -41.0822) (52.338, -41.3015) (52.5897, -41.2996) knots 0 0 0 0 1 1 1 1
  spline S626 degree 3 poles (52.5897, -41.2996) (52.8325, -41.2976) (53.0989, -41.0815) (53.1018, -40.8893) knots 0 0 0 0 1 1 1 1
  spline S627 degree 3 poles (53.1018, -40.8893) (53.1047, -40.6912) (52.8372, -40.4597) (52.587, -40.4568) knots 0 0 0 0 1 1 1 1
  spline S628 degree 3 poles (51.9604, -37.6254) (51.7066, -37.6224) (51.4203, -37.8508) (51.4221, -38.0516) knots 0 0 0 0 1 1 1 1
  spline S629 degree 3 poles (51.4221, -38.0516) (51.4238, -38.2509) (51.7115, -38.4702) (51.9631, -38.4683) knots 0 0 0 0 1 1 1 1
  spline S630 degree 3 poles (51.9631, -38.4683) (52.206, -38.4663) (52.4724, -38.2502) (52.4752, -38.058) knots 0 0 0 0 1 1 1 1
  spline S631 degree 3 poles (52.4752, -38.058) (52.4781, -37.8599) (52.2106, -37.6284) (51.9604, -37.6254) knots 0 0 0 0 1 1 1 1
  spline S632 degree 3 poles (54.1397, -37.4958) (53.886, -37.4928) (53.5997, -37.7212) (53.6014, -37.9219) knots 0 0 0 0 1 1 1 1
  spline S633 degree 3 poles (53.6014, -37.9219) (53.6031, -38.1212) (53.8908, -38.3406) (54.1425, -38.3386) knots 0 0 0 0 1 1 1 1
  spline S634 degree 3 poles (54.1425, -38.3386) (54.3853, -38.3367) (54.6517, -38.1205) (54.6546, -37.9283) knots 0 0 0 0 1 1 1 1
  spline S635 degree 3 poles (54.6546, -37.9283) (54.6575, -37.7302) (54.39, -37.4987) (54.1397, -37.4958) knots 0 0 0 0 1 1 1 1
  spline S636 degree 3 poles (17.6677, -44.0931) (17.5885, -43.8923) (17.6297, -43.6335) (17.9117, -43.5025) knots 0 0 0 0 1 1 1 1
  line L128 (17.9117, -43.5025) -> (19.6163, -42.711)
  spline S637 degree 3 poles (19.6163, -42.711) (19.7803, -42.6348) (20.0852, -42.6643) (20.2019, -42.8221) knots 0 0 0 0 1 1 1 1
  spline S638 degree 2 poles (20.2019, -42.8221) (23.7005, -47.312) (24.9271, -48.6047) knots 0 0 0 1 1 1
  spline S639 degree 3 poles (24.9271, -48.6047) (25.9764, -49.7103) (27.2417, -50.4391) (28.7329, -50.5141) knots 0 0 0 0 1 1 1 1
  spline S640 degree 2 poles (28.7329, -50.5141) (31.8378, -50.6703) (41.7412, -50.045) knots 0 0 0 1 1 1
  spline S641 degree 3 poles (41.7412, -50.045) (42.6105, -50.0155) (42.4081, -47.6671) (41.7397, -47.6689) knots 0 0 0 0 1 1 1 1
  line L129 (41.7397, -47.6689) -> (35.5069, -47.6858)
  spline S642 degree 3 poles (35.5069, -47.6858) (35.2579, -47.6864) (35.1777, -47.5931) (35.1749, -47.2604) knots 0 0 0 0 1 1 1 1
  line L130 (35.1749, -47.2604) -> (35.1589, -45.3744)
  spline S643 degree 3 poles (35.1589, -45.3744) (35.1566, -45.1049) (35.0917, -44.9984) (34.7542, -44.9959) knots 0 0 0 0 1 1 1 1
  line L131 (34.7542, -44.9959) -> (31.0523, -44.9664)
  spline S644 degree 3 poles (31.0523, -44.9664) (30.6887, -44.9636) (30.6099, -44.8519) (30.6155, -44.3354) knots 0 0 0 0 1 1 1 1
  line L132 (30.6155, -44.3354) -> (30.6935, -37.1303)
  spline S645 degree 3 poles (30.6935, -37.1303) (30.7035, -36.1994) (28.6199, -35.689) (28.5346, -33.5102) knots 0 0 0 0 1 1 1 1
  spline S646 degree 3 poles (28.5346, -33.5102) (28.4025, -30.1388) (31.3951, -29.8238) (31.3932, -28.7937) knots 0 0 0 0 1 1 1 1
  line L133 (31.3932, -28.7937) -> (31.3884, -26.1847)
  spline S647 degree 3 poles (31.3884, -26.1847) (31.388, -25.975) (31.5497, -25.9389) (31.6727, -25.9368) knots 0 0 0 0 1 1 1 1
  line L134 (31.6727, -25.9368) -> (34.4913, -25.8858)
  spline S648 degree 3 poles (34.4913, -25.8858) (34.6153, -25.8836) (34.7393, -25.9776) (34.7411, -26.1085) knots 0 0 0 0 1 1 1 1
  line L135 (34.7411, -26.1085) -> (34.7575, -27.3402)
  spline S649 degree 3 poles (34.7575, -27.3402) (34.76, -27.8151) (34.967, -27.902) (35.2844, -27.9224) knots 0 0 0 0 1 1 1 1
  spline S650 degree 2 poles (35.2844, -27.9224) (37.2723, -27.9013) (37.2868, -27.914) knots 0 0 0 1 1 1
  spline S651 degree 3 poles (37.2868, -27.914) (37.476, -27.9098) (37.4998, -27.8058) (37.5031, -27.7023) knots 0 0 0 0 1 1 1 1
  line L136 (37.5031, -27.7023) -> (37.5131, -27.3857)
  spline S652 degree 3 poles (37.5131, -27.3857) (37.5084, -27.1689) (37.6238, -27.1706) (37.8051, -27.1702) knots 0 0 0 0 1 1 1 1
  line L137 (37.8051, -27.1702) -> (41.0154, -27.1618)
  spline S653 degree 3 poles (41.0154, -27.1618) (41.2607, -27.1611) (41.4955, -27.1239) (41.5277, -26.7442) knots 0 0 0 0 1 1 1 1
  line L138 (41.5277, -26.7442) -> (41.5037, -22.0656)
  spline S654 degree 3 poles (41.5037, -22.0656) (41.5015, -21.6343) (41.5551, -21.5748) (41.9553, -21.5813) knots 0 0 0 0 1 1 1 1
  spline S655 degree 2 poles (41.9553, -21.5813) (43.9778, -21.4588) (44.5822, -21.7523) knots 0 0 0 1 1 1
  spline S656 degree 3 poles (44.5822, -21.7523) (44.8796, -21.8967) (47.386, -25.03) (48.117, -26.7341) knots 0 0 0 0 1 1 1 1
  spline S657 degree 3 poles (48.117, -26.7341) (48.7968, -28.3188) (49.0204, -28.6069) (50.6474, -28.5648) knots 0 0 0 0 1 1 1 1
  spline S658 degree 2 poles (50.6474, -28.5648) (51.905, -28.5312) (55.6953, -28.4491) knots 0 0 0 1 1 1
  spline S659 degree 3 poles (55.6953, -28.4491) (56.1552, -28.4448) (56.3401, -28.5594) (56.3598, -29.0042) knots 0 0 0 0 1 1 1 1
  line L139 (56.3598, -29.0042) -> (56.4984, -32.1267)
  spline S660 degree 3 poles (56.4984, -32.1267) (56.495, -32.7827) (56.8532, -32.9883) (57.3288, -32.9429) knots 0 0 0 0 1 1 1 1
  line L140 (57.3288, -32.9429) -> (58.4232, -32.9134)
  spline S661 degree 3 poles (58.4232, -32.9134) (58.9816, -32.8839) (59.3493, -33.0759) (59.3673, -33.7523) knots 0 0 0 0 1 1 1 1
  line L141 (59.3673, -33.7523) -> (59.7313, -47.3943)
  spline S662 degree 3 poles (59.7313, -47.3943) (59.7393, -47.6608) (59.7972, -47.8571) (59.4421, -47.8749) knots 0 0 0 0 1 1 1 1
  line L142 (59.4421, -47.8749) -> (57.5604, -47.9697)
  spline S663 degree 3 poles (57.5604, -47.9697) (57.3015, -47.9823) (57.1434, -48.1751) (57.1473, -48.4479) knots 0 0 0 0 1 1 1 1
  line L143 (57.1473, -48.4479) -> (57.1964, -51.8655)
  spline S664 degree 3 poles (57.1964, -51.8655) (57.2044, -52.4317) (57.1037, -52.5249) (56.7432, -52.5441) knots 0 0 0 0 1 1 1 1
  line L144 (56.7432, -52.5441) -> (48.405, -52.9882)
  spline S665 degree 3 poles (48.405, -52.9882) (47.6336, -53.0303) (46.3815, -55.2618) (43.9146, -55.3499) knots 0 0 0 0 1 1 1 1
  spline S666 degree 3 poles (43.9146, -55.3499) (41.4654, -55.4374) (41.2131, -53.4186) (40.5831, -53.4553) knots 0 0 0 0 1 1 1 1
  spline S667 degree 2 poles (40.5831, -53.4553) (22.9283, -54.6237) (21.736, -54.3768) knots 0 0 0 1 1 1
  spline S668 degree 2 poles (21.736, -54.3768) (20.9507, -54.2143) (17.6688, -44.0982) knots 0 0 0 1 1 1
  line L145 (17.6688, -44.0982) -> (17.6677, -44.0931)
  spline S669 degree 3 poles (15.3621, -42.4125) (15.2581, -44.2071) (19.2027, -57.8957) (24.3714, -60.2393) knots 0 0 0 0 1 1 1 1
  spline S670 degree 3 poles (24.3714, -60.2393) (26.0618, -61.0058) (28.7417, -61.2698) (29.6435, -60.8371) knots 0 0 0 0 1 1 1 1
  spline S671 degree 3 poles (29.6435, -60.8371) (37.8199, -56.9138) (43.4149, -58.1646) (51.8713, -58.0302) knots 0 0 0 0 1 1 1 1
  spline S672 degree 3 poles (51.8713, -58.0302) (59.516, -57.9086) (62.8527, -50.0146) (63.1445, -44.2408) knots 0 0 0 0 1 1 1 1
  spline S673 degree 3 poles (63.1445, -44.2408) (63.7798, -31.6714) (58.1767, -23.4257) (51.5097, -20.3069) knots 0 0 0 0 1 1 1 1
  spline S674 degree 3 poles (51.5097, -20.3069) (41.2773, -15.5202) (26.6816, -19.883) (23.1701, -29.7543) knots 0 0 0 0 1 1 1 1
  spline S675 degree 3 poles (23.1701, -29.7543) (22.3709, -32.001) (22.6133, -34.4085) (21.5017, -36.3646) knots 0 0 0 0 1 1 1 1